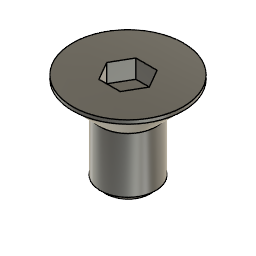
M3 Parametric FHCS (Autodesk Fusion 360 design; units mm, degrees)
part number: M3x5mm FHCS
Autodesk Fusion 360 part; units mm, degrees
note: some values were not read from the file. Set by a fixed rule: which sketch regions a step uses.
sketch "Sketch1" plane through (0, 0, 0) normal (1, 0, 0) x (0, 1, 0)
  line L0 (0, 5) -> (3, 5)
  line L1 (3, 5) -> (3, 4.8)
  line L2 (3, 4.8) -> (1.5, 3.3)
  line L3 (1.5, 3.3) -> (1.5, 0.3)
  line L4 (1.2, 0) -> (0, 0)
  line L5 (0, 0) -> (0, 5)
  line L6 (1.5, 0.3) -> (1.2, 0)
  point P0 (1.5, 0)
  dimension "d1" = 1.5
  dimension "d3" = 5
  dimension "d4" = 1.7
  dimension "d5" = 135
  dimension "d6" = 3
  dimension "d9" = 0.3
  dimension "d10" = 0.3
  constraint horizontal L0
  constraint perpendicular L0 L1
  constraint perpendicular L0 L3
  constraint perpendicular L3 L4
  constraint vertical L5
  constraint coincident L0.start L5.end
  constraint coincident L4.end L5
  constraint coincident L4.end L5.start
  constraint coincident L3 P0
  constraint coincident L4 P0
  measures "d1" distance of L3 L5
  measures "d3" distance of L0 L4
  measures "d4" distance of L0 L2.end
  measures "d5" angle of L2 L3
  measures "d6" distance of L1 L5
  measures "d9" distance of L3.end P0
  measures "d10" distance of L4.start P0
revolve "Revolve1" add sketch "Sketch1" angle 360 about axis through (0, 0, 0) along (0, 0, 1)
sketch "Sketch2" plane through (0, 0, 5) normal (0, 0, 1) x (-1, 0, 0)
  circle A0 centre (0, 0) radius 3
  line L0 (0.5774, -1) -> (1.1547, 0)
  line L1 (1.1547, 0) -> (0.5774, 1)
  line L2 (0.5774, 1) -> (-0.5774, 1)
  line L3 (-0.5774, 1) -> (-1.1547, 0)
  line L4 (-1.1547, 0) -> (-0.5774, -1)
  line L5 (-0.5774, -1) -> (0.5774, -1)
  dimension "d11" = 1
  constraint coincident A0.centre origin
  constraint horizontal L5
  measures "d11" distance of A0.centre L5
extrude "Extrude1" cut sketch "Sketch2" against normal blind 1 contours L0 L1 L2 L3 L4 L5
equation "d1 = ( 3 / 2 ) * 1 mm"
equation "d3 = Length"
equation "d4 = Head_Length"
equation "d6 = Head_Diameter / 2"
equation "Length = 5 mm"
equation "d10 = d9"
equation "Head_Diameter = 6 mm"
equation "Head_Length = 1.7 mm"
